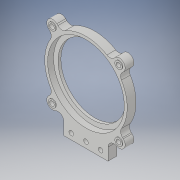
# Autodesk Inventor part: outer_bearing_holder_new
Saved by Autodesk Inventor 2019.4 (Build 234330000, 330)
## iProperties
Created: 2019-08-03
Part Number: outer_bearing_holder_new
Material: Generic
Document SubType Name: Modeling
Designer: cdi
Density: 1 g/cm^3
Appearance: Default
Author: cdi
Autodesk Inventor part; units mm, degrees
ref_plane "YZ Plane" through (0, 0, 0) normal (1, 0, 0) x (0, 1, 0)
ref_plane "XZ Plane" through (0, 0, 0) normal (0, 1, 0) x (-1, 0, 0)
ref_plane "XY Plane" through (0, 0, 0) normal (0, 0, 1) x (1, 0, 0)
sketch "Sketch1" plane through (0, 0, 0) normal (0, 0, 1) x (1, 0, 0)
  circle A0 centre (0, 0) radius 28
  circle A1 centre (0, 0) radius 23
  dimension "d0" = 56
  dimension "d1" = 46
  constraints: 2 centre point, 2 coincident
  measures "d0" diameter of A0
  measures "d1" diameter of A1
extrude "Extrusion1" add sketch "Sketch1" along normal blind 6
sketch "Sketch2" plane through (0, 0, 6) normal (0, 0, 1) x (1, 0, 0)
  circle A0 centre (0, 0) radius 26.025
  dimension "d4" = 52.05
  constraints: 1 centre point, 1 coincident
  measures "d4" diameter of A0
extrude "Extrusion2" cut sketch "Sketch2" against normal blind 4.05
sketch "Sketch3" plane through (0, 0, 0) normal (0, 0, -1) x (-1, 0, 0)
  line L0 (0, 0) -> (-40.3791, 40.3791)
  line L1 (0, 0) -> (-48.4868, 0)
  circle A0 centre (-22.6274, 22.6274) radius 1.5
  arc A1 (-19.7033, 25.3568) -> (-25.4558, 19.799) centre (-22.6274, 22.6274) ccw
  line L2 (-25.4558, 19.799) -> (-22.4243, 16.7675)
  line L3 (-19.7033, 25.3568) -> (-16.8842, 22.3366)
  circle A2 centre (0, 0) radius 28 projected
  dimension "d7" = 45
  dimension "d8" = 3
  dimension "d9" = 4
  dimension "d23" = 32
  constraints: 8 end point, 4 point on circle, 2 centre point, 2 tangent, 1 coincident, 1 horizontal, 1 point on line
  measures "d7" angle of L0 L1
  measures "d8" diameter of A0
  measures "d9" radius of A1
  measures "d23" distance of L0.start A0.centre
extrude "Extrusion3" add sketch "Sketch3" against normal up to surface (6 mm away) contours A2 L2 A1 L0 A0 | L0 A0 A1 L3 A2 | A0 L0 | L0 A0
sketch "Sketch4" plane through (0, 0, 0) normal (0, 0, -1) x (-1, 0, 0)
  arc A0 (-19.7033, 25.3568) -> (-25.4558, 19.799) centre (-22.6274, 22.6274) ccw projected
  point P0 (0, 0)
hole "Hole1" at (22.6274, 22.6274, 0) direction (0, 0, 1) diameter 3.1 depth 10 countersink diameter 6.5 countersink angle 90
fillet "Fillet1" radius 4 2 edges at (22.4243, 16.7675, 3) (16.8842, 22.3366, 3)
sketch "Sketch5" plane through (0, 0, 6) normal (0, 0, 1) x (1, 0, 0)
  arc A0 (25.4558, 19.799) -> (19.799, 25.4558) centre (22.6274, 22.6274) ccw projected
  circle A1 centre (22.6274, 22.6274) radius 2.5
  circle A2 centre (22.6274, 22.6274) radius 1.55 projected
  point P0 (0, 0)
  dimension "d24" = 5
  constraints: 1 centre point, 1 coincident
  measures "d24" diameter of A1
extrude "Extrusion4" add sketch "Sketch5" along normal blind 0.5
pattern_circular "Circular Pattern2" count 4 over 360 about axis through (0, 0, 0) along (0, 0, 1) of "Extrusion3", "Hole1", "Fillet1", "Extrusion4"
sketch "Sketch6" plane through (0, 0, 0) normal (0, 0, -1) x (-1, 0, 0)
  line L0 (-15, -38) -> (15, -38)
  line L1 (15, -38) -> (15, -30)
  line L2 (15, -30) -> (-15, -30)
  line L3 (-15, -30) -> (-15, -38)
  point P0 (0, 0)
  dimension "d30" = 15
  dimension "d31" = 30
  dimension "d32" = 30
  dimension "d53" = 38
  constraints: 8 end point, 2 parallel, 1 horizontal, 1 perpendicular
  measures "d30" distance from line of point (0, 0) L1
  measures "d31" distance of L0.start L0.end
  measures "d32" distance from line of point (0, 0) L2
  measures "d53" distance from line of point (0, 0) L0
extrude "Extrusion5" add sketch "Sketch6" against normal up to surface (6 mm away)
sketch "Sketch7" plane through (-15, -30, 0) normal (0, 1, 0) x (1, 0, 0)
  line L0 (0, -6) -> (30, -6) projected
  line L1 (30, 0) -> (30, -6) projected
  line L2 (0, 0) -> (30, 0) projected
  line L3 (0, 0) -> (0, -6) projected
  point P0 (15, 0)
extrude "Extrusion6" add sketch "Sketch7" along normal up to surface
fillet "Fillet2" radius 4 2 edges at (-15, -23.7599, 3) (15, -23.7668, 3)
sketch "Sketch8" plane through (0, 0, 0) normal (0, 0, -1) x (-1, 0, 0)
  line L0 (-15, -38) -> (15, -38) projected
  line L1 (-15, -34) -> (15, -34)
  circle A0 centre (0, -34) radius 1.5
  point P0 (0, 0)
  dimension "d38" = 4
  dimension "d39" = 3
  constraints: 2 end point, 1 centre point, 1 midpoint, 1 parallel
  measures "d38" distance between parallel lines of L0 L1
  measures "d39" diameter of A0
hole "Hole2" at (0, -34, 0) direction (0, 0, 1) diameter 3.1 depth 10 countersink diameter 6.5 countersink angle 90
pattern_linear "Rectangular Pattern1" count 2 spacing 10 along (-1, 0, 0) count 2 spacing 10 along (1, 0, 0) of "Hole2"
body "Solid1"
